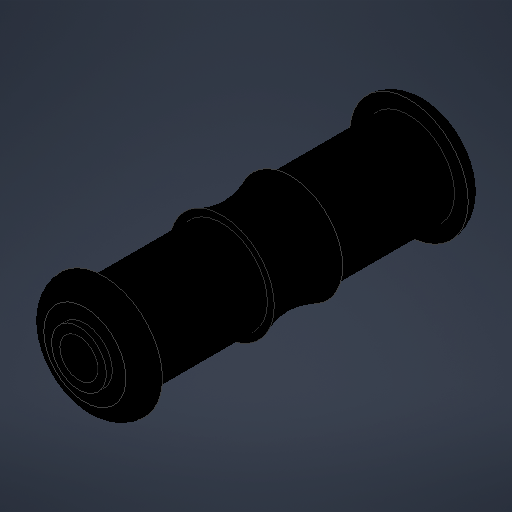
# Autodesk Inventor part: Dribbler Roller Seperator
Saved by Autodesk Inventor 2026.1 (Build 301233020, 233B)
## iProperties
Created: 2025-12-15
Part Number: Dribbler Roller Seperator
Material: Generic
Document SubType Name: Modeling
Designer: Bahaa
Density: 1 g/cm^3
Appearance: Default
Author: Bahaa
Autodesk Inventor part; units mm, degrees
ref_plane "YZ Plane" through (0, 0, 0) normal (1, 0, 0) x (0, 1, 0)
ref_plane "XZ Plane" through (0, 0, 0) normal (0, 1, 0) x (-1, 0, 0)
ref_plane "XY Plane" through (0, 0, 0) normal (0, 0, 1) x (1, 0, 0)
sketch "Sketch1" plane through (0, 0, 0) normal (0, 1, 0) x (-1, 0, 0)
  circle A0 centre (0, 0) radius 2.0875
  circle A1 centre (0, 0) radius 5
  circle A2 centre (0, 0) radius 5.75
  circle A3 centre (0, 0) radius 6.5
  circle A4 centre (0, 0) radius 3
  dimension "d0" = 4.175
  dimension "d1" = 10
  dimension "d4" = 11.5
  dimension "d7" = 13
  dimension "d16" = 6
  constraints: 5 centre point, 5 coincident
  measures "d0" diameter of A0
  measures "d1" diameter of A1
  measures "d4" diameter of A2
  measures "d7" diameter of A3
  measures "d16" diameter of A4
extrude "Extrusion1" add sketch "Sketch1" along normal blind 37.5 contours A1 | A4
ref_plane "Work Plane1" through (0, 18.75, 0) normal (0, -1, 0) x (1, 0, 0)
extrude "Extrusion2" add sketch "Sketch1" along normal mid plane 7.5 from surface at 18.75 contours A2
extrude "Extrusion3" add sketch "Sketch1" along normal blind 2 contours A2 | A3
extrude "Extrusion4" add sketch "Sketch1" against normal blind 2 from surface at 37.5 contours A1 | A2 | A3 | A4
fillet "Fillet1" radius 2 2 edges at (6.5, 0, 0) (6.5, 37.5, 0)
sketch "Sketch2" plane through (0, 0, 0) normal (0, 0, 1) x (1, 0, 0)
  line L0 (5.75, 22.5) -> (-5.75, 22.5) projected
  line L1 (5.75, 15) -> (-5.75, 15) projected
  arc A0 (5.75, 22.5) -> (5.75, 15) centre (13.9315, 18.75) ccw
  line L2 (5.75, 15) -> (5.75, 22.5) projected
  line L3 (0, 15.281) -> (0, 22.5)
  point P0 (0, 0)
  dimension "d15" = 9
  constraints: 2 end point, 2 point on circle, 1 centre point, 1 midpoint
  measures "d15" radius of A0
revolve "Revolution1" cut sketch "Sketch2" angle 360 about axis through (0, 15.281, 0) along (0, 1, 0)
extrude "Extrusion5" add sketch "Sketch1" against normal blind 0.65 contours A4
mirror "Mirror1" about plane through (0, 18.75, 0) normal (0, -1, 0) of "Extrusion5"
body "Solid1"
